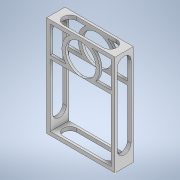
# Autodesk Inventor part: box rim big
Saved by Autodesk Inventor 2021 (Build 250183000, 183)
## iProperties
Created: 2021-06-29
Part Number: box rim big
Material: Generic
Document SubType Name: Modeling
Designer: newic
Density: 1 g/cm^3
Appearance: Default
Author: newic
Autodesk Inventor part; units mm, degrees
ref_plane "YZ Plane" through (0, 0, 0) normal (1, 0, 0) x (0, 1, 0)
ref_plane "XZ Plane" through (0, 0, 0) normal (0, 1, 0) x (-1, 0, 0)
ref_plane "XY Plane" through (0, 0, 0) normal (0, 0, 1) x (1, 0, 0)
sketch "Sketch1" plane through (0, 0, 0) normal (1, 0, 0) x (0, 1, 0)
  line L0 (0, 0) -> (0, -31.75)
  line L1 (0, 0) -> (173.355, 0)
  line L2 (0, 0) -> (173.355, 0)
  line L3 (173.355, 0) -> (173.355, -31.75)
  line L4 (173.355, -31.75) -> (0, -31.75)
  line L5 (0, -31.75) -> (0, 0)
  line L6 (0, -15.875) -> (6.35, -15.875)
  line L7 (173.355, -15.875) -> (167.005, -15.875)
  arc A0 (155.0924, -27.7876) -> (155.0924, -3.9624) centre (155.0924, -15.875) ccw
  line L8 (155.0924, -3.9624) -> (30.9626, -3.9624)
  line L9 (30.9626, -27.7876) -> (155.0924, -27.7876)
  arc A1 (30.9626, -3.9624) -> (30.9626, -27.7876) centre (30.9626, -15.875) ccw
  dimension "d0" = 31.75
  dimension "d1" = 173.355
  dimension "d2" = 6.35
  dimension "d3" = 6.35
  constraints: 20 end point, 5 horizontal, 4 point on circle, 3 tangent, 2 centre point, 2 midpoint, 2 parallel, 1 perpendicular, 1 vertical
  measures "d0" distance of L0.start L0.end
  measures "d1" distance of L0.start L1.end
  measures "d2" distance of L6.start L6.end
  measures "d3" distance of L7.start L7.end
extrude "Extrusion1" add sketch "Sketch1" against normal blind 118.11
sketch "Sketch2" plane through (0, 0, 0) normal (0, 0, 1) x (1, 0, 0)
  line L0 (0, 173.355) -> (0, 0) projected
  line L1 (0, 173.355) -> (-118.11, 173.355) projected
  line L2 (-118.11, 0) -> (-118.11, 173.355) projected
  line L3 (0, 0) -> (-118.11, 0) projected
  line L4 (-6.35, 6.35) -> (-6.35, 167.005)
  line L5 (-6.35, 167.005) -> (-111.76, 167.005)
  line L6 (-111.76, 167.005) -> (-111.76, 6.35)
  line L7 (-111.76, 6.35) -> (-6.35, 6.35)
  dimension "d9" = 6.35
  constraints: 8 end point, 3 other
  measures "d9" distance between parallel lines of L0 L4
extrude "Extrusion2" cut sketch "Sketch2" against normal blind 118.11 contours L7 L6 L5 L4
sketch "Sketch3" plane through (0, 0, 0) normal (0, 0, 1) x (1, 0, 0)
  point P0 (0, 0)
sketch "Sketch4" plane through (0, 0, 0) normal (0, 0, 1) x (1, 0, 0)
  line L0 (-111.76, 167.005) -> (-6.35, 167.005) projected
  circle A0 centre (-59.055, 140.6525) radius 26.3525
  line L1 (-111.76, 30.9626) -> (-111.76, 155.0924) projected
  line L2 (-111.76, 114.3) -> (-6.35, 114.3)
  line L3 (-6.35, 114.3) -> (-6.35, 167.005)
  line L4 (-6.35, 167.005) -> (-111.76, 167.005)
  line L5 (-111.76, 167.005) -> (-111.76, 114.3)
  point P0 (0, 0)
  point P1 (-59.055, 167.005)
  point P2 (-59.055, 114.3)
  constraints: 8 end point, 2 parallel, 1 centre point, 1 horizontal, 1 perpendicular, 1 point on line
extrude "Extrusion3" add sketch "Sketch4" against normal blind 31.75 contours L0 A0 L2 L1 L5 | L0 L3 L2 A0
sketch "Sketch5" plane through (0, 0, 0) normal (1, 0, 0) x (0, 0, -1)
  line L0 (0, 173.355) -> (0, 0) projected
  line L1 (0, 0) -> (31.75, 0) projected
  line L2 (31.75, 0) -> (31.75, 173.355) projected
  line L3 (31.75, 173.355) -> (0, 173.355) projected
  arc A0 (27.7876, 155.0924) -> (3.9624, 155.0924) centre (15.875, 155.0924) ccw projected
  line L4 (27.7876, 155.0924) -> (27.7876, 30.9626) projected
  arc A1 (3.9624, 30.9626) -> (27.7876, 30.9626) centre (15.875, 30.9626) ccw projected
  line L5 (3.9624, 30.9626) -> (3.9624, 155.0924) projected
extrude "Extrusion4" cut sketch "Sketch5" against normal through all contours L4 A1 L5 A0
sketch "Sketch6" plane through (0, 0, -31.75) normal (0, -1, 0) x (1, 0, 0)
  line L0 (-118.11, 3.9624) -> (-118.11, 27.7876) projected
  line L1 (0, 27.7876) -> (0, 3.9624) projected
  line L2 (-81.0991, 27.7876) -> (-118.11, 27.7876) projected
  line L3 (-99.6046, 27.7876) -> (-18.2626, 27.7876)
  line L4 (-6.35, 3.9624) -> (-59.055, 3.9624) projected
  line L5 (-18.2626, 3.9624) -> (-99.6046, 3.9624)
  line L6 (-81.0991, 3.9624) -> (-118.11, 3.9624) projected
  line L7 (0, 0) -> (0, 31.75) projected
  line L8 (0, 15.875) -> (-12.7, 15.875)
  line L9 (-118.11, 0) -> (-118.11, 31.75) projected
  line L10 (-118.11, 15.875) -> (-105.41, 15.875)
  arc A0 (-24.6126, 3.9624) -> (-24.6126, 27.7876) centre (-24.6126, 15.875) ccw
  arc A1 (-93.4974, 27.7876) -> (-93.4974, 3.9624) centre (-93.4974, 15.875) ccw
  dimension "d21" = 12.7
  dimension "d22" = 12.7
  constraints: 8 end point, 5 point on line, 4 midpoint, 4 point on circle, 2 centre point, 2 horizontal, 1 collinear
  measures "d21" distance of L8.start L8.end
  measures "d22" distance of L10.start L10.end
extrude "Extrusion5" cut sketch "Sketch6" against normal blind 31.75 contours A1 L2 L3 A0 L4 L5
sketch "Sketch7" plane through (0, 173.355, 0) normal (0, 1, 0) x (1, 0, 0)
  line L0 (-24.6126, 3.9624) -> (-93.4974, 3.9624) projected
  line L1 (-93.4974, 27.7876) -> (-24.6126, 27.7876) projected
  arc A0 (-93.4974, 27.7876) -> (-93.4974, 3.9624) centre (-93.4974, 15.875) ccw projected
  arc A1 (-24.6126, 3.9624) -> (-24.6126, 27.7876) centre (-24.6126, 15.875) ccw projected
  point P0 (0, 0)
extrude "Extrusion6" cut sketch "Sketch7" against normal blind 31.75
sketch "Sketch8" plane through (0, 0, 0) normal (0, 0, 1) x (1, 0, 0)
  line L0 (-111.76, 6.35) -> (-111.76, 114.3) projected
  line L1 (-111.76, 114.3) -> (-59.055, 114.3) projected
  circle A0 centre (-59.055, 140.6525) radius 26.3525 projected
  line L2 (-59.055, 114.3) -> (-6.35, 114.3) projected
  line L3 (-6.35, 114.3) -> (-6.35, 6.35) projected
  line L4 (-6.35, 6.35) -> (-111.76, 6.35) projected
  line L5 (0, 173.355) -> (0, 0) projected
  line L6 (0, 173.355) -> (-118.11, 173.355) projected
  line L7 (-118.11, 0) -> (-118.11, 173.355) projected
  line L8 (0, 0) -> (-118.11, 0) projected
  line L9 (-59.055, 120.65) -> (-118.11, 120.65)
  line L10 (-118.11, 120.65) -> (-118.11, 0)
  line L11 (-118.11, 0) -> (0, 0)
  line L12 (0, 0) -> (0, 120.65)
  line L13 (0, 120.65) -> (-59.055, 120.65)
  line L14 (-111.76, 167.005) -> (-6.35, 167.005)
  line L15 (-6.35, 167.005) -> (-6.35, 6.35)
  line L16 (-6.35, 6.35) -> (-111.76, 6.35)
  line L17 (-111.76, 6.35) -> (-111.76, 167.005)
  circle A1 centre (-59.055, 140.6525) radius 32.7025
  point P0 (-39.6901, 167.005)
  point P1 (-33.1831, 120.65)
  point P2 (-6.35, 120.65)
  point P3 (-84.9269, 120.65)
  point P4 (-78.4199, 167.005)
  point P5 (-111.76, 120.65)
  dimension "d27" = 6.35
  dimension "d28" = 6.35
  dimension "d29" = 6.35
  constraints: 18 end point, 1 centre point, 1 vertical alignment, 7 other
  measures "d27" distance between parallel lines of L1 L9
  measures "d28" distance between parallel lines of L7 L17
extrude "Extrusion7" cut sketch "Sketch8" against normal through all contours L17 L14 A1 L9 | L13 A1 L14 L15
body "Solid1"
